GT2_20Pulley_v1 (Autodesk Fusion 360 design; units mm, degrees)
Autodesk Fusion 360 part; units mm, degrees
note: some values were not read from the file. Chosen so that the rebuilt part matches the saved one: which face or edge a step refers to; which sketch regions a step uses.
sketch "Sketch5" plane through (0, 0, 0) normal (0, 1, 0) x (1, 0, 0)
  line L0 (0, -3.12) -> (0, -8)
  line L1 (0, -8) -> (7.6, -8)
  line L2 (7.6, -8) -> (7.6, -6.12)
  line L3 (7.6, -6.12) -> (14.9, -6.12)
  line L4 (14.9, -6.12) -> (14.9, -8)
  line L5 (14.9, -8) -> (16, -8)
  line L6 (16, -8) -> (16, -4.22)
  line L7 (16, -4.22) -> (15.9, -4.12)
  line L8 (15.9, -4.12) -> (16, -4.02)
  line L9 (16, -4.02) -> (16, -3.12)
  line L10 (16, -3.12) -> (0, -3.12)
  line L11 (15.9, -4.12) -> (8.0872, -4.12) construction
  dimension "d24" = 90
  dimension "d25" = 3
  dimension "d26" = 3.12
  dimension "d30" = 1
  dimension "d31" = 7.3
  dimension "d32" = 0.1
  dimension "d33" = 7.6
  dimension "d34" = 1.1
  dimension "d35" = 8
  dimension "d36" = 8
  constraint vertical L0
  constraint horizontal L1
  constraint horizontal L3
  constraint vertical L2
  constraint vertical L4
  constraint horizontal L10
  constraint vertical L9
  constraint vertical L6
  constraint horizontal L5
  constraint coincident origin L0
  constraint collinear L6 L9
  constraint horizontal L11
  constraint symmetric L7 L8 L11
  measures "d24" angle of L7 L8
  measures "d25" distance of L3 L10
  measures "d26" distance of origin L10
  measures "d30" distance of L7.end L10
  measures "d31" horizontal distance of L2.end L3.end
  measures "d32" distance of L7.end L9
  measures "d33" horizontal distance of L0.end L1.end
  measures "d34" distance of L4.end L5.end
  measures "d35" distance of origin L1
  measures "d36" distance of origin L5
revolve "Revolve1" add sketch "Sketch5" angle 360 about axis through (1.75, 0, 0) along (1, 0, 0)
sketch "Sketch4" plane through (14.9, 0, 0) normal (-1, 0, 0) x (0, 0, 1)
  circle A0 centre (0, 0) radius 8
  circle A1 centre (0, 0) radius 6.125
  line L0 (0, 0) -> (0, 6.125) construction
  circle A2 centre (0, 0) radius 5.375 construction
  circle A3 centre (0, 0) radius 5.93 construction
  arc A4 (-0.4989, 5.6868) -> (0, 5.375) centre (0, 5.93) ccw
  arc A5 (-0.5855, 5.9553) -> (-0.4989, 5.6868) centre (0.4, 6.125) ccw
  arc A6 (-0.5855, 5.9553) -> (-0.7517, 6.0787) centre (-0.7333, 5.9298) ccw
  arc A7 (0.7517, 6.0787) -> (0.5855, 5.9553) centre (0.7333, 5.9298) ccw
  arc A8 (0.4989, 5.6868) -> (0.5855, 5.9553) centre (-0.4, 6.125) ccw
  arc A9 (0, 5.375) -> (0.4989, 5.6868) centre (0, 5.93) ccw
  circle A10 centre (0, 0) radius 8
  circle A11 centre (0, 0) radius 6.12
  dimension "d10" = 6.125
  dimension "d12" = 0.75
  dimension "d14" = 0.4
  dimension "d16" = 1
  dimension "d18" = 0.555
  dimension "d19" = 0.15
  constraint coincident A0.centre A1.centre
  constraint vertical L0
  constraint coincident A4.centre L0
  constraint tangent A2 A4
  constraint concentric A2 A3
  constraint coincident A4.centre A3
  constraint tangent A1 A6
  constraint tangent A5 A6
  constraint tangent A4 A5
  constraint coincident L0 A4.end
  constraint coincident A1 A6.end
  constraint symmetric L0 A4 A9
  constraint symmetric L0 A5 A8
  constraint symmetric L0 A4.end A9.start
  constraint symmetric L0 A4.start A8.start
  constraint symmetric L0 A6 A7
  constraint symmetric L0 A5.start A7.end
  constraint symmetric L0 A6.end A7.start
  measures "d10" vertical distance of A0.centre L0.end
  measures "d12" distance of A1 A2
  measures "d14" distance of L0 A5.centre
  measures "d16" radius of A5
  measures "d18" radius of A4
  measures "d19" radius of A6
extrude "Extrude5" cut sketch "Sketch4" along normal blind 7.3 contours A1 A4 A5 A6 A7 A8 A9 A11 picked at (0, 5.8716)
pattern_circular "C-Pattern1" count 20 over 360 about axis through (1.75, 0, 0) along (1, 0, 0) of "Extrude5"
hole "Hole1" at (3, 0, 8) direction (0, 0, -1) diameter 3 depth 8 tip angle 118
hole "Hole2" at (3, 8, 0) direction (0, -1, 0) diameter 3 depth 5.5 tip angle 118
chamfer "Chamfer1" distance 0.5 angle 45 4 edges at (3, 7.8581, 1.5) (3, 7.8581, -1.5) (3, 1.5, 7.8581) (3, -1.5, 7.8581)
delete_face "Fläche löschen1" 3 faces at (1.8808, -1.4479, 7.698) (1.1736, 0.159, 7.8317) (4.8315, -0.0809, 7.8329)
delete_face "Fläche löschen2" 1 faces at (4.4937, -0.1373, 6.3704)
move_face "Fläche verschieben1" to x (1, 0, 0) y (0, 1, 0) z (0, 0, 1) at (2, 0, 0) 2 faces at (2.0986, 5.8968, 1.1989) (1.3769, 7.7864, 0.8514)
move_face "Flächen versetzen1" offset -2 1 faces at (0, 0.3974, 6.3435)
named bodies: "GT2-20T-6Bore"
